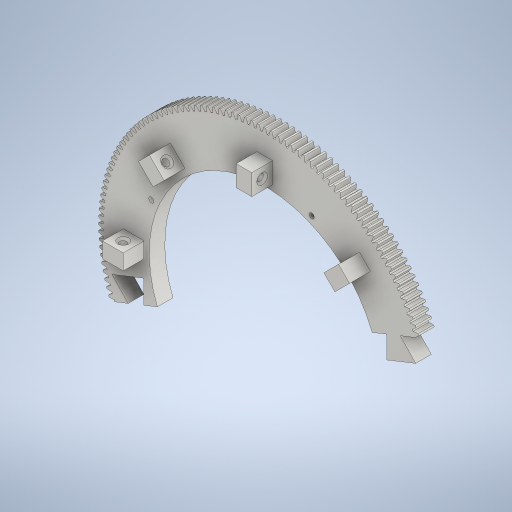
# Autodesk Inventor part: BearingGearMk2
Saved by Autodesk Inventor 2023 (Build 270158000, 158)
## iProperties
CustomPartVersion: 1
Created: 2023-04-03
Part Number: BearingGearMk2
Material: Steel
Document SubType Name: Modeling
Designer: czapa
Categories: <?xml version="1.0" encoding="UTF-16"?> <MemberInstance><Categories><FamilyTemplate><FamilyTemplateParameter ValueType="xs:double" Id="1" ObjectReferenceKey="da_z" ObjectType="kUserParameterObject"/><FamilyTemplateParameter ValueType="xs:double" Id="2" ObjectReferenceKey="da_b" ObjectType="kUserParameterObject"/><FamilyTemplateParameter ValueType="xs:double" Id="3" ObjectReferenceKey="da_beta" ObjectType="kUserParameterObject"/><FamilyTemplateParameter ValueType="xs:double" Id="4" ObjectReferenceKey="da_da" ObjectType="kUserParameterObject"/><FamilyTemplateParameter ValueType="xs:double" Id="5" ObjectReferenceKey="da_aw" ObjectType="kUserParameterObject"/><FamilyTemplateParameter ValueType="xs:string" Id="6" ObjectReferenceKey="EAIAABAAAACIAQAAAAAAAIAAAAAAAAAA" ObjectType="83910656" SubObjectId="SurfaceGeometry"/></FamilyTemplate><ParamToTemplateMap><ParamToTemplate CategoryParameter="//CategoryParameter[@InternalName='046C89C9-8512-4d59-83FE-43B91F4F132A']" TemplateParameter="1"/><ParamToTemplate CategoryParameter="//CategoryParameter[@InternalName='2552DF32-E462-4b46-AEBF-C6C7768E72AC']" TemplateParameter="2"/><ParamToTemplate CategoryParameter="//CategoryParameter[@InternalName='C9EE641D-15FC-4fae-A226-E94C4372FDD7']" TemplateParameter="3"/><ParamToTemplate><ParamToTemplate CategoryParameter="//CategoryParameter[@InternalName='00B6519A-459B-49c7-AD84-2E56D39A5744']" ConstantValue="-1.000000"/></ParamToTemplate><ParamToTemplate><ParamToTemplate CategoryParameter="//CategoryParameter[@InternalName='04B31F0E-C7A6-4894-AA32-9629BEFACF47']" ConstantValue="1.000000"/></ParamToTemplate><ParamToTemplate><ParamToTemplate CategoryParameter="//CategoryParameter[@InternalName='43CBEC2E-7847-49e7-A936-2F7889FCB2D9']" ConstantValue="0.250000"/></ParamToTemplate><ParamToTemplate><ParamToTemplate CategoryParameter="//CategoryParameter[@InternalName='B1EFC894-105D-4ebd-86BF-FA20ED196853']" ConstantValue="0.350000"/></ParamToTemplate><ParamToTemplate><ParamToTemplate CategoryParameter="//CategoryParameter[@InternalName='51175063-3D10-4879-93E8-6246FE8B403D']" ConstantValue="2060000000.000000"/></ParamToTemplate><ParamToTemplate><ParamToTemplate CategoryParameter="//CategoryParameter[@InternalName='A3A52E27-4454-46a9-B0BD-C932399B70AF']" ConstantValue="0.300000"/></ParamToTemplate><ParamToTemplate><ParamToTemplate CategoryParameter="//CategoryParameter[@InternalName='91B76062-C214-41d9-B1B9-14D2AB99603D']" ConstantValue="0.200000"/></ParamToTemplate><ParamToTemplate><ParamToTemplate CategoryParameter="//CategoryParameter[@InternalName='374E806E-8B8A-4dda-A9AA-1039D6500AD2']" ConstantValue="5.000000"/></ParamToTemplate><ParamToTemplate><ParamToTemplate CategoryParameter="//CategoryParameter[@InternalName='2D373A89-B862-43d6-8D0B-0CBF12AB9F6C']" ConstantValue="0.349066"/></ParamToTemplate><ParamToTemplate CategoryParameter="//CategoryParameter[@InternalName='37777632-D6A2-4fac-9D53-DB8ACD95C989']" TemplateParameter="4"/><ParamToTemplate CategoryParameter="//CategoryParameter[@InternalName='FD1017F1-B727-4f7e-9707-0F86F1FF9423']" TemplateParameter="5"/><ParamToTemplate><ParamToTemplate CategoryParameter="//CategoryParameter[@InternalName='9E1B4470-B2D3-4ff1-B813-535BB4CDF51A']" ConstantValue="3520000.000000"/></ParamToTemplate><ParamToTemplate><ParamToTemplate CategoryParameter="//CategoryParameter[@InternalName='F8452263-BFF6-458c-9FB1-07C4B99E95CD']" ConstantValue="11400000.000000"/></ParamToTemplate><ParamToTemplate><ParamToTemplate CategoryParameter="//CategoryParameter[@InternalName='3E3BB259-FD49-497f-8171-6EBC954A3479']" ConstantValue="2.000000"/></ParamToTemplate><ParamToTemplate CategoryParameter="//CategoryParameter[@InternalName='27C3BAF2-7550-4e4b-AE2C-0DB134B7D9B7']" TemplateParameter="6"/></ParamToTemplateMap><Category DisplayName="Gear" InternalName="DC85795E-93AB-48d5-8EEE-5A27447B64BD" Mnemonic="Gear"><CategoryParameter DisplayName="z" InternalName="046C89C9-8512-4d59-83FE-43B91F4F132A" Mnemonic="z"/><CategoryParameter DisplayName="b" InternalName="2552DF32-E462-4b46-AEBF-C6C7768E72AC" Mnemonic="b"/><CategoryParameter DisplayName="||b|" InternalName="C9EE641D-15FC-4fae-A226-E94C4372FDD7" Mnemonic="beta"/><CategoryParameter DisplayName="x" InternalName="00B6519A-459B-49c7-AD84-2E56D39A5744" Mnemonic="x"/><CategoryParameter DisplayName="a*" InternalName="04B31F0E-C7A6-4894-AA32-9629BEFACF47" Mnemonic="a"/><CategoryParameter DisplayName="c*" InternalName="43CBEC2E-7847-49e7-A936-2F7889FCB2D9" Mnemonic="c"/><CategoryParameter DisplayName="r|.f|*" InternalName="B1EFC894-105D-4ebd-86BF-FA20ED196853" Mnemonic="rf"/><CategoryParameter DisplayName="E" InternalName="51175063-3D10-4879-93E8-6246FE8B403D" Mnemonic="E"/><CategoryParameter DisplayName="||m|" InternalName="A3A52E27-4454-46a9-B0BD-C932399B70AF" Mnemonic="mi"/><Category DisplayName="SpurGear" InternalName="26C5A22E-A91E-4dfd-A3B3-23CCAFAE1764" Mnemonic="SpurGear"><CategoryParameter DisplayName="m" InternalName="91B76062-C214-41d9-B1B9-14D2AB99603D" Mnemonic="m"/><CategoryParameter DisplayName="P" InternalName="374E806E-8B8A-4dda-A9AA-1039D6500AD2" Mnemonic="PP"/><CategoryParameter DisplayName="||a|" InternalName="2D373A89-B862-43d6-8D0B-0CBF12AB9F6C" Mnemonic="alpha"/><CategoryParameter DisplayName="d|.a|" InternalName="37777632-D6A2-4fac-9D53-DB8ACD95C989" Mnemonic="da"/><CategoryParameter DisplayName="a|.w|" InternalName="FD1017F1-B727-4f7e-9707-0F86F1FF9423" Mnemonic="aw"/><CategoryParameter DisplayName="||s||.Flim|" InternalName="9E1B4470-B2D3-4ff1-B813-535BB4CDF51A" Mnemonic="sFlim"/><CategoryParameter DisplayName="||s||.Hlim|" InternalName="F8452263-BFF6-458c-9FB1-07C4B99E95CD" Mnemonic="sHlim"/><CategoryParameter DisplayName="type" InternalName="3E3BB259-FD49-497f-8171-6EBC954A3479" Mnemonic="type"/><CategoryParameter DisplayName="PitchDiameter" InternalName="27C3BAF2-7550-4e4b-AE2C-0DB134B7D9B7" Mnemonic="IDS_PITCHDIAM"/></Category></Category></Categories></MemberInstance>
Density: 1 g/cm^3
Appearance: Steel
Author: czapa
Autodesk Inventor part; units mm, degrees
(part 1 of 2)
ref_plane "YZ Plane" through (0, 0, 0) normal (1, 0, 0) x (0, 1, 0)
ref_plane "XZ Plane" through (0, 0, 0) normal (0, 1, 0) x (-1, 0, 0)
ref_plane "XY Plane" through (0, 0, 0) normal (0, 0, 1) x (1, 0, 0)
sketch "Sketch1" plane through (0, 0, 0) normal (0, 0, 1) x (1, 0, 0)
  circle A0 centre (0, 0) radius 160
  dimension "d0" = 320
  constraints: 1 centre point
  measures "d0" diameter of A0
extrude "Extrusion1" add sketch "Sketch1" along normal blind 15
ref_plane "Work Plane2" through (0, 0, 7.5) normal (0, 0, 1) x (1, 0, 0)
sketch "Sketch2" plane through (0, 0, 0) normal (0, 0, -1) x (-1, 0, 0)
  circle A0 centre (0, 0) radius 160 projected
  circle A1 centre (0, 0) radius 160
  dimension "d3" = 320
  constraints: 1 centre point, 1 coincident
  measures "d3" diameter of A1
surface extrude "Pitch Diameter" sketch "Sketch2" against normal through all shown no curves A1
ref_plane "Work Plane8" through (0, 0, 0) normal (0.9998072, 0.0196337, 0) x (0, 0, 1)
ref_plane "Work Plane9" through (0, 0, 0) normal (1, 0, 0) x (0, 1, 0)
spur gear teeth "Spur Gear" teeth 160 pitch diameter 320 tip diameter 320 root diameter 311 face width 20 start plane through (0, 0, 0) normal (0, 0, -1) x (-1, 0, 0)
sketch "Sketch3" plane through (0, 0, 15) normal (0, 0, 1) x (1, 0, 0)
  circle A0 centre (0, 0) radius 125
  circle A1 centre (0, 0) radius 111.25
  dimension "d49" = 250
  dimension "d50" = 222.5
  constraints: 2 centre point, 2 coincident
  measures "d49" diameter of A0
  measures "d50" diameter of A1
extrude "Extrusion2" cut sketch "Sketch3" against normal blind 15 contours A1
sketch "Sketch7" plane through (0, 0, 15) normal (0, 0, 1) x (1, 0, 0)
  line L0 (0, 116.25) -> (7.5, 116.25)
  line L1 (7.5, 116.25) -> (7.5, 136.25)
  line L2 (7.5, 116.25) -> (-7.5, 116.25)
  line L3 (-7.5, 116.25) -> (-7.5, 136.25)
  line L4 (-7.5, 136.25) -> (7.5, 136.25)
  line L5 (7.5, 136.25) -> (7.5, 116.25)
  line L6 (0, 0) -> (111.25, 0) construction
  circle A0 centre (0, 0) radius 111.25 projected
  point P0 (7.5, 136.25)
  point P1 (0, 111.25)
  dimension "d75" = 7.5
  dimension "d76" = 20
  dimension "d77" = 15
  dimension "d78" = 20
  dimension "d110" = 5
  constraints: 14 end point, 2 horizontal, 2 parallel, 2 perpendicular, 1 midpoint, 1 point on circle
  measures "d75" distance of L0.start L0.end
  measures "d76" distance of L0.end L1.end
  measures "d77" distance of L3.end L4.end
  measures "d78" distance of L2.end L3.end
  measures "d110" distance of A0.end point (0, 116.25)
extrude "Extrusion4" add sketch "Sketch7" along normal blind 20 contours L2 L3 L4 L1 L0
sketch "Sketch8" plane through (7.5, 116.25, 15) normal (1, 0, 0) x (0, 0, -1)
  line L0 (-20, 20) -> (-20, 0) projected
  line L1 (-20, 10) -> (-10, 10)
  line L2 (0, 20) -> (-20, 20) projected
  circle A0 centre (-10, 10) radius 3.25
  point P0 (15, -116.25)
  dimension "d81" = 6.5
  constraints: 2 end point, 1 centre point, 1 coincident, 1 midpoint, 1 parallel
  measures "d81" diameter of A0
extrude "Extrusion5" cut sketch "Sketch8" against normal blind 20
chamfer "Chamfer1" distance 2 angle 45 2 edges at (-7.5, 126.25, 28.25) (7.5, 126.25, 28.25)
pattern_circular "Circular Pattern3" count 8 over 360 about axis through (0, 0, 15) along (0, 0, -1) of "Extrusion4", "Extrusion5", "Chamfer1"
sketch "Sketch10" plane through (0, 0, 15) normal (0, 0, 1) x (1, 0, 0)
  circle A0 centre (0, 0) radius 118.125
  line L0 (0, 0) -> (45.2045, 109.1333)
  line L1 (0, 0) -> (118.125, 0) construction
  dimension "d111" = 67.5
  constraints: 4 end point, 2 coincident, 1 equal length, 1 horizontal, 3 other
  measures "d111" angle of L1 L0
hole "Hole2" at (45.2045, 109.1333, 15) direction (0, 0, -1) diameter 5 end through all
pattern_circular "Circular Pattern4" count 4 over 360 about axis through (0, 0, 15) along (0, 0, -1) of "Hole2"
sketch "Sketch11" plane through (0, 0, 15) normal (0, 0, 1) x (1, 0, 0)
  circle A0 centre (0, 0) radius 111.25 projected
  line L0 (0, 0) -> (111.25, 0) construction
  arc A1 (148.1195, 60.503) -> (147.5184, 61.9542) centre (0, 0) ccw projected
  line L1 (0, 0) -> (144.524, 57.3853)
  line L2 (0, 0) -> (3.1399, -7.9077)
  line L3 (0, 0) -> (-144.524, -57.3853)
  arc A2 (-144.524, -57.3853) -> (-148.1195, -60.503) centre (-126.4791, -81.8277) ccw projected
  line L4 (-144.524, -57.3853) -> (-123.9607, -49.2203)
  line L5 (-123.9607, -49.2203) -> (-116.5799, -67.8086)
  line L6 (-116.5799, -67.8086) -> (-102.6387, -62.2731)
  line L7 (-102.6387, -62.2731) -> (-117.4002, -46.6154)
  line L8 (-123.9607, -49.2203) -> (-131.3414, -30.632)
  line L9 (-117.4002, -25.0965) -> (-117.4002, -46.6154)
  line L10 (-117.4002, -46.6154) -> (-116.4708, -46.2464)
  line L11 (-117.4002, -25.0965) -> (-117.7692, -24.1671)
  line L12 (-117.7692, -24.1671) -> (-114.0516, -22.6909)
  line L13 (-116.4708, -23.6515) -> (-116.4708, -46.2464)
  line L14 (-145.2826, -36.1676) -> (-130.5212, -51.8253)
  line L15 (-145.2826, -36.1676) -> (-145.6517, -35.2382)
  line L16 (-145.6517, -35.2382) -> (-149.3693, -36.7143)
  line L17 (-146.9501, -35.7538) -> (-131.4506, -52.1943)
  line L18 (-145.6517, -35.2382) -> (-117.7692, -24.1671)
  line L19 (-116.5799, -67.8086) -> (-130.5212, -73.3442)
  line L20 (-130.5212, -73.3442) -> (-130.5212, -51.8253)
  line L21 (123.9607, 49.2203) -> (131.3414, 30.632)
  line L22 (131.3414, 30.632) -> (117.4002, 25.0965)
  line L23 (117.4002, 25.0965) -> (117.4002, 46.6154)
  line L24 (145.2826, 36.1676) -> (130.5212, 51.8253)
  line L25 (131.3414, 30.632) -> (145.2826, 36.1676)
  circle A3 centre (-109.1333, 45.2045) radius 2.5 projected
  circle A4 centre (-45.2045, -109.1333) radius 2.5 projected
  circle A5 centre (109.1333, -45.2045) radius 2.5 projected
  circle A6 centre (45.2045, 109.1333) radius 2.5 projected
  line L26 (-101.6466, 91.04) -> (-91.04, 101.6466) projected
  line L27 (-91.04, 101.6466) -> (-76.8979, 87.5045) projected
  line L28 (-76.8979, 87.5045) -> (-87.5045, 76.8979) projected
  line L29 (-87.5045, 76.8979) -> (-101.6466, 91.04) projected
  line L30 (-136.25, -7.5) -> (-136.25, 7.5) projected
  line L31 (-136.25, 7.5) -> (-116.25, 7.5) projected
  line L32 (-116.25, 7.5) -> (-116.25, -7.5) projected
  line L33 (-116.25, -7.5) -> (-136.25, -7.5) projected
  line L34 (-91.04, -101.6466) -> (-101.6466, -91.04) projected
  line L35 (-101.6466, -91.04) -> (-87.5045, -76.8979) projected
  line L36 (-87.5045, -76.8979) -> (-76.8979, -87.5045) projected
  line L37 (-76.8979, -87.5045) -> (-91.04, -101.6466) projected
  line L38 (7.5, -136.25) -> (-7.5, -136.25) projected
  line L39 (-7.5, -136.25) -> (-7.5, -116.25) projected
  line L40 (-7.5, -116.25) -> (7.5, -116.25) projected
  line L41 (7.5, -116.25) -> (7.5, -136.25) projected
  line L42 (101.6466, -91.04) -> (91.04, -101.6466) projected
  line L43 (91.04, -101.6466) -> (76.8979, -87.5045) projected
  line L44 (76.8979, -87.5045) -> (87.5045, -76.8979) projected
  line L45 (87.5045, -76.8979) -> (101.6466, -91.04) projected
  line L46 (136.25, 7.5) -> (136.25, -7.5) projected
  line L47 (136.25, -7.5) -> (116.25, -7.5) projected
  line L48 (116.25, -7.5) -> (116.25, 7.5) projected
  line L49 (116.25, 7.5) -> (136.25, 7.5) projected
  line L50 (91.04, 101.6466) -> (101.6466, 91.04) projected
  line L51 (101.6466, 91.04) -> (87.5045, 76.8979) projected
  line L52 (87.5045, 76.8979) -> (76.8979, 87.5045) projected
  line L53 (76.8979, 87.5045) -> (91.04, 101.6466) projected
  line L54 (-7.5, 136.25) -> (7.5, 136.25) projected
  line L55 (7.5, 136.25) -> (7.5, 116.25) projected
  line L56 (7.5, 116.25) -> (-7.5, 116.25) projected
  line L57 (-7.5, 116.25) -> (-7.5, 136.25) projected
  circle A7 centre (0, 0) radius 111.25 projected
  arc A8 (-7.0663, 159.8439) -> (-8.3923, 155.2734) centre (21.3596, 149.1191) ccw projected
  arc A9 (-8.3923, 155.2734) -> (-9.9163, 155.1835) centre (0, 0) ccw projected
  arc A10 (-9.9163, 155.1835) -> (-11.7703, 159.5665) centre (-38.7386, 145.575) ccw projected
  arc A11 (-11.7703, 159.5665) -> (-13.3363, 159.4432) centre (0, 0) ccw projected
  arc A12 (-13.3363, 159.4432) -> (-14.4819, 154.8242) centre (15.4887, 149.8427) ccw projected
  arc A13 (-14.4819, 154.8242) -> (-16.0011, 154.6745) centre (0, 0) ccw projected
  arc A14 (-16.0011, 154.6745) -> (-18.0258, 158.9814) centre (-44.424, 143.9419) ccw projected
  arc A15 (-18.0258, 158.9814) -> (-19.5857, 158.7967) centre (0, 0) ccw projected
  arc A16 (-19.5857, 158.7967) -> (-20.5491, 154.1363) centre (9.594, 150.3353) ccw projected
  arc A17 (-20.5491, 154.1363) -> (-22.0613, 153.9271) centre (0, 0) ccw projected
  arc A18 (-22.0613, 153.9271) -> (-24.2535, 158.1511) centre (-50.0409, 142.0868) ccw projected
  arc A19 (-24.2535, 158.1511) -> (-25.8049, 157.9054) centre (0, 0) ccw projected
  arc A20 (-25.8049, 157.9054) -> (-26.5846, 153.2107) centre (3.6845, 150.5961) ccw projected
  arc A21 (-26.5846, 153.2107) -> (-28.0874, 152.9423) centre (0, 0) ccw projected
  arc A22 (-28.0874, 152.9423) -> (-30.4438, 157.077) centre (-55.5806, 140.0127) ccw projected
  arc A23 (-30.4438, 157.077) -> (-31.9844, 156.7705) centre (0, 0) ccw projected
  arc A24 (-31.9844, 156.7705) -> (-32.5791, 152.0488) centre (-2.2308, 150.6246) ccw projected
  arc A25 (-32.5791, 152.0488) -> (-34.0702, 151.7217) centre (0, 0) ccw projected
  arc A26 (-34.0702, 151.7217) -> (-36.5871, 155.7607) centre (-61.0346, 137.7226) ccw projected
  arc A27 (-36.5871, 155.7607) -> (-38.1145, 155.394) centre (0, 0) ccw projected
  arc A28 (-38.1145, 155.394) -> (-38.5234, 150.6526) centre (-8.1425, 150.4209) ccw projected
  arc A29 (-38.5234, 150.6526) -> (-40.0005, 150.2671) centre (0, 0) ccw projected
  arc A30 (-40.0005, 150.2671) -> (-42.674, 154.2042) centre (-66.3945, 135.2203) ccw projected
  arc A31 (-42.674, 154.2042) -> (-44.1859, 153.7778) centre (0, 0) ccw projected
  arc A32 (-44.1859, 153.7778) -> (-44.4083, 149.024) centre (-14.0418, 149.9853) ccw projected
  arc A33 (-44.4083, 149.024) -> (-45.8692, 148.5809) centre (0, 0) ccw projected
  arc A34 (-45.8692, 148.5809) -> (-48.6952, 152.4099) centre (-71.6521, 132.5094) ccw projected
  arc A35 (-48.6952, 152.4099) -> (-50.1891, 151.9245) centre (0, 0) ccw projected
  arc A36 (-50.1891, 151.9245) -> (-50.2247, 147.1657) centre (-19.9193, 149.3183) ccw projected
  arc A37 (-50.2247, 147.1657) -> (-51.6671, 146.6655) centre (0, 0) ccw projected
  arc A38 (-51.6671, 146.6655) -> (-54.6412, 150.3806) centre (-76.7991, 129.5942) ccw projected
  arc A39 (-54.6412, 150.3806) -> (-56.1149, 149.837) centre (0, 0) ccw projected
  arc A40 (-56.1149, 149.837) -> (-55.9637, 145.0804) centre (-25.7662, 148.4212) ccw projected
  arc A41 (-55.9637, 145.0804) -> (-57.3853, 144.524) centre (0, 0) ccw projected
  arc A42 (-57.3853, 144.524) -> (-60.503, 148.1195) centre (-81.8277, 126.4791) ccw projected
  arc A43 (-60.503, 148.1195) -> (-61.9542, 147.5184) centre (0, 0) ccw projected
  arc A44 (-61.9542, 147.5184) -> (-61.6164, 142.7714) centre (-31.5733, 147.2952) ccw projected
  arc A45 (-61.6164, 142.7714) -> (-63.015, 142.1596) centre (0, 0) ccw projected
  arc A46 (-63.015, 142.1596) -> (-66.2715, 145.63) centre (-86.7302, 123.1691) ccw projected
  arc A47 (-66.2715, 145.63) -> (-67.698, 144.9723) centre (0, 0) ccw projected
  arc A48 (-67.698, 144.9723) -> (-67.174, 140.2423) centre (-37.3317, 145.9421) ccw projected
  arc A49 (-67.174, 140.2423) -> (-68.5476, 139.5761) centre (0, 0) ccw projected
  arc A50 (-68.5476, 139.5761) -> (-71.9378, 142.9159) centre (-91.4989, 119.6691) ccw projected
  arc A51 (-71.9378, 142.9159) -> (-73.3374, 142.2028) centre (0, 0) ccw projected
  arc A52 (-73.3374, 142.2028) -> (-72.6281, 137.4969) centre (-43.0326, 144.3639) ccw projected
  arc A53 (-72.6281, 137.4969) -> (-73.9745, 136.7773) centre (0, 0) ccw projected
  arc A54 (-73.9745, 136.7773) -> (-77.4932, 139.9814) centre (-96.1266, 115.9846) ccw projected
  arc A55 (-77.4932, 139.9814) -> (-78.8637, 139.2139) centre (0, 0) ccw projected
  arc A56 (-78.8637, 139.2139) -> (-77.9702, 134.5396) centre (-48.6671, 142.5632) ccw projected
  arc A57 (-77.9702, 134.5396) -> (-79.2873, 133.7676) centre (0, 0) ccw projected
  arc A58 (-79.2873, 133.7676) -> (-82.9291, 136.8312) centre (-100.606, 112.1213) ccw projected
  arc A59 (-82.9291, 136.8312) -> (-84.2684, 136.0104) centre (0, 0) ccw projected
  arc A60 (-84.2684, 136.0104) -> (-83.1921, 131.3747) centre (-54.2266, 140.5426) ccw projected
  arc A61 (-83.1921, 131.3747) -> (-84.4779, 130.5517) centre (0, 0) ccw projected
  arc A62 (-84.4779, 130.5517) -> (-88.2371, 133.4699) centre (-104.9303, 108.0851) ccw projected
  arc A63 (-88.2371, 133.4699) -> (-89.5432, 132.5972) centre (0, 0) ccw projected
  arc A64 (-89.5432, 132.5972) -> (-88.2857, 128.0073) centre (-59.7025, 138.3053) ccw projected
  arc A65 (-88.2857, 128.0073) -> (-89.5382, 127.1344) centre (0, 0) ccw projected
  arc A66 (-89.5382, 127.1344) -> (-93.4091, 129.9028) centre (-109.0928, 103.8822) ccw projected
  arc A67 (-93.4091, 129.9028) -> (-94.6799, 128.9795) centre (0, 0) ccw projected
  arc A68 (-94.6799, 128.9795) -> (-93.2432, 124.4426) centre (-65.0863, 135.8548) ccw projected
  arc A69 (-93.2432, 124.4426) -> (-94.4604, 123.5212) centre (0, 0) ccw projected
  arc A70 (-94.4604, 123.5212) -> (-98.4371, 126.1354) centre (-113.0871, 99.5191) ccw projected
  arc A71 (-98.4371, 126.1354) -> (-99.6706, 125.163) centre (0, 0) ccw projected
  arc A72 (-99.6706, 125.163) -> (-98.0569, 120.6859) centre (-70.3698, 133.1948) ccw projected
  arc A73 (-98.0569, 120.6859) -> (-99.237, 119.7174) centre (0, 0) ccw projected
  arc A74 (-99.237, 119.7174) -> (-103.3132, 122.1736) centre (-116.907, 95.0026) ccw projected
  arc A75 (-103.3132, 122.1736) -> (-104.5077, 121.1534) centre (0, 0) ccw projected
  arc A76 (-104.5077, 121.1534) -> (-102.7194, 116.7432) centre (-75.5447, 130.3294) ccw projected
  arc A77 (-102.7194, 116.7432) -> (-103.8606, 115.7291) centre (0, 0) ccw projected
  arc A78 (-103.8606, 115.7291) -> (-108.0301, 118.0233) centre (-120.5467, 90.3396) ccw projected
  arc A79 (-108.0301, 118.0233) -> (-109.1835, 116.9571) centre (0, 0) ccw projected
  arc A80 (-109.1835, 116.9571) -> (-107.2236, 112.6204) centre (-80.6032, 127.263) ccw projected
  arc A81 (-107.2236, 112.6204) -> (-108.324, 111.5623) centre (0, 0) ccw projected
  arc A82 (-108.324, 111.5623) -> (-112.5804, 113.6911) centre (-124.0004, 85.5374) ccw projected
  arc A83 (-112.5804, 113.6911) -> (-113.6911, 112.5804) centre (0, 0) ccw projected
  arc A84 (-113.6911, 112.5804) -> (-111.5623, 108.324) centre (-85.5374, 124.0004) ccw projected
  arc A85 (-111.5623, 108.324) -> (-112.6204, 107.2236) centre (0, 0) ccw projected
  arc A86 (-112.6204, 107.2236) -> (-116.9571, 109.1835) centre (-127.263, 80.6032) ccw projected
  arc A87 (-116.9571, 109.1835) -> (-118.0233, 108.0301) centre (0, 0) ccw projected
  arc A88 (-118.0233, 108.0301) -> (-115.7291, 103.8606) centre (-90.3396, 120.5467) ccw projected
  arc A89 (-115.7291, 103.8606) -> (-116.7432, 102.7194) centre (0, 0) ccw projected
  arc A90 (-116.7432, 102.7194) -> (-121.1534, 104.5077) centre (-130.3294, 75.5447) ccw projected
  arc A91 (-121.1534, 104.5077) -> (-122.1736, 103.3132) centre (0, 0) ccw projected
  arc A92 (-122.1736, 103.3132) -> (-119.7174, 99.237) centre (-95.0026, 116.907) ccw projected
  arc A93 (-119.7174, 99.237) -> (-120.6859, 98.0569) centre (0, 0) ccw projected
  arc A94 (-120.6859, 98.0569) -> (-125.163, 99.6706) centre (-133.1948, 70.3698) ccw projected
  arc A95 (-125.163, 99.6706) -> (-126.1354, 98.4371) centre (0, 0) ccw projected
  arc A96 (-126.1354, 98.4371) -> (-123.5212, 94.4604) centre (-99.5191, 113.0871) ccw projected
  arc A97 (-123.5212, 94.4604) -> (-124.4426, 93.2432) centre (0, 0) ccw projected
  arc A98 (-124.4426, 93.2432) -> (-128.9795, 94.6799) centre (-135.8548, 65.0863) ccw projected
  arc A99 (-128.9795, 94.6799) -> (-129.9028, 93.4091) centre (0, 0) ccw projected
  arc A100 (-129.9028, 93.4091) -> (-127.1344, 89.5382) centre (-103.8822, 109.0928) ccw projected
  arc A101 (-127.1344, 89.5382) -> (-128.0073, 88.2857) centre (0, 0) ccw projected
  arc A102 (-128.0073, 88.2857) -> (-132.5972, 89.5432) centre (-138.3053, 59.7025) ccw projected
  arc A103 (-132.5972, 89.5432) -> (-133.4699, 88.2371) centre (0, 0) ccw projected
  arc A104 (-133.4699, 88.2371) -> (-130.5517, 84.4779) centre (-108.0851, 104.9303) ccw projected
  arc A105 (-130.5517, 84.4779) -> (-131.3747, 83.1921) centre (0, 0) ccw projected
  arc A106 (-131.3747, 83.1921) -> (-136.0104, 84.2684) centre (-140.5426, 54.2266) ccw projected
  arc A107 (-136.0104, 84.2684) -> (-136.8312, 82.9291) centre (0, 0) ccw projected
  arc A108 (-136.8312, 82.9291) -> (-133.7676, 79.2873) centre (-112.1213, 100.606) ccw projected
  arc A109 (-133.7676, 79.2873) -> (-134.5396, 77.9702) centre (0, 0) ccw projected
  arc A110 (-134.5396, 77.9702) -> (-139.2139, 78.8637) centre (-142.5632, 48.6671) ccw projected
  arc A111 (-139.2139, 78.8637) -> (-139.9814, 77.4932) centre (0, 0) ccw projected
  arc A112 (-139.9814, 77.4932) -> (-136.7773, 73.9745) centre (-115.9846, 96.1266) ccw projected
  arc A113 (-136.7773, 73.9745) -> (-137.4969, 72.6281) centre (0, 0) ccw projected
  arc A114 (-137.4969, 72.6281) -> (-142.2028, 73.3374) centre (-144.3639, 43.0326) ccw projected
  arc A115 (-142.2028, 73.3374) -> (-142.9159, 71.9378) centre (0, 0) ccw projected
  arc A116 (-142.9159, 71.9378) -> (-139.5761, 68.5476) centre (-119.6691, 91.4989) ccw projected
  arc A117 (-139.5761, 68.5476) -> (-140.2423, 67.174) centre (0, 0) ccw projected
  arc A118 (-140.2423, 67.174) -> (-144.9723, 67.698) centre (-145.9421, 37.3317) ccw projected
  arc A119 (-144.9723, 67.698) -> (-145.63, 66.2715) centre (0, 0) ccw projected
  arc A120 (-145.63, 66.2715) -> (-142.1596, 63.015) centre (-123.1691, 86.7302) ccw projected
  arc A121 (-142.1596, 63.015) -> (-142.7714, 61.6164) centre (0, 0) ccw projected
  arc A122 (-142.7714, 61.6164) -> (-147.5184, 61.9542) centre (-147.2952, 31.5733) ccw projected
  arc A123 (-147.5184, 61.9542) -> (-148.1195, 60.503) centre (0, 0) ccw projected
  arc A124 (-148.1195, 60.503) -> (-144.524, 57.3853) centre (-126.4791, 81.8277) ccw projected
  arc A125 (-144.524, 57.3853) -> (-145.0804, 55.9637) centre (0, 0) ccw projected
  arc A126 (-145.0804, 55.9637) -> (-149.837, 56.1149) centre (-148.4212, 25.7662) ccw projected
  arc A127 (-149.837, 56.1149) -> (-150.3806, 54.6412) centre (0, 0) ccw projected
  arc A128 (-150.3806, 54.6412) -> (-146.6655, 51.6671) centre (-129.5942, 76.7991) ccw projected
  arc A129 (-146.6655, 51.6671) -> (-147.1657, 50.2247) centre (0, 0) ccw projected
  arc A130 (-147.1657, 50.2247) -> (-151.9245, 50.1891) centre (-149.3183, 19.9193) ccw projected
  arc A131 (-151.9245, 50.1891) -> (-152.4099, 48.6952) centre (0, 0) ccw projected
  arc A132 (-152.4099, 48.6952) -> (-148.5809, 45.8692) centre (-132.5094, 71.6521) ccw projected
  arc A133 (-148.5809, 45.8692) -> (-149.024, 44.4083) centre (0, 0) ccw projected
  arc A134 (-149.024, 44.4083) -> (-153.7778, 44.1859) centre (-149.9853, 14.0418) ccw projected
  arc A135 (-153.7778, 44.1859) -> (-154.2042, 42.674) centre (0, 0) ccw projected
  arc A136 (-154.2042, 42.674) -> (-150.2671, 40.0005) centre (-135.2203, 66.3945) ccw projected
  arc A137 (-150.2671, 40.0005) -> (-150.6526, 38.5234) centre (0, 0) ccw projected
  arc A138 (-150.6526, 38.5234) -> (-155.394, 38.1145) centre (-150.4209, 8.1425) ccw projected
  arc A139 (-155.394, 38.1145) -> (-155.7607, 36.5871) centre (0, 0) ccw projected
  arc A140 (-155.7607, 36.5871) -> (-151.7217, 34.0702) centre (-137.7226, 61.0346) ccw projected
  arc A141 (-151.7217, 34.0702) -> (-152.0488, 32.5791) centre (0, 0) ccw projected
  arc A142 (-152.0488, 32.5791) -> (-156.7705, 31.9844) centre (-150.6246, 2.2308) ccw projected
  arc A143 (-156.7705, 31.9844) -> (-157.077, 30.4438) centre (0, 0) ccw projected
  arc A144 (-157.077, 30.4438) -> (-152.9423, 28.0874) centre (-140.0127, 55.5806) ccw projected
  arc A145 (-152.9423, 28.0874) -> (-153.2107, 26.5846) centre (0, 0) ccw projected
  arc A146 (-153.2107, 26.5846) -> (-157.9054, 25.8049) centre (-150.5961, -3.6845) ccw projected
  arc A147 (-157.9054, 25.8049) -> (-158.1511, 24.2535) centre (0, 0) ccw projected
  arc A148 (-158.1511, 24.2535) -> (-153.9271, 22.0613) centre (-142.0868, 50.0409) ccw projected
  arc A149 (-153.9271, 22.0613) -> (-154.1363, 20.5491) centre (0, 0) ccw projected
  arc A150 (-154.1363, 20.5491) -> (-158.7967, 19.5857) centre (-150.3353, -9.594) ccw projected
  arc A151 (-158.7967, 19.5857) -> (-158.9814, 18.0258) centre (0, 0) ccw projected
  arc A152 (-158.9814, 18.0258) -> (-154.6745, 16.0011) centre (-143.9419, 44.424) ccw projected
  arc A153 (-154.6745, 16.0011) -> (-154.8242, 14.4819) centre (0, 0) ccw projected
  arc A154 (-154.8242, 14.4819) -> (-159.4432, 13.3363) centre (-149.8427, -15.4887) ccw projected
  arc A155 (-159.4432, 13.3363) -> (-159.5665, 11.7703) centre (0, 0) ccw projected
  arc A156 (-159.5665, 11.7703) -> (-155.1835, 9.9163) centre (-145.575, 38.7386) ccw projected
  arc A157 (-155.1835, 9.9163) -> (-155.2734, 8.3923) centre (0, 0) ccw projected
  arc A158 (-155.2734, 8.3923) -> (-159.8439, 7.0663) centre (-149.1191, -21.3596) ccw projected
  arc A159 (-159.8439, 7.0663) -> (-159.9056, 5.4967) centre (0, 0) ccw projected
  arc A160 (-159.9056, 5.4967) -> (-155.4532, 3.8162) centre (-146.9836, 32.9935) ccw projected
  arc A161 (-155.4532, 3.8162) -> (-155.4831, 2.2898) centre (0, 0) ccw projected
  arc A162 (-155.4831, 2.2898) -> (-159.9981, 0.7854) centre (-148.1656, -27.1975) ccw projected
  arc A163 (-159.9981, 0.7854) -> (-159.9981, -0.7854) centre (0, 0) ccw projected
  arc A164 (-159.9981, -0.7854) -> (-155.4831, -2.2898) centre (-148.1656, 27.1975) ccw projected
  arc A165 (-155.4831, -2.2898) -> (-155.4532, -3.8162) centre (0, 0) ccw projected
  arc A166 (-155.4532, -3.8162) -> (-159.9056, -5.4967) centre (-146.9836, -32.9935) ccw projected
  arc A167 (-159.9056, -5.4967) -> (-159.8439, -7.0663) centre (0, 0) ccw projected
  arc A168 (-159.8439, -7.0663) -> (-155.2734, -8.3923) centre (-149.1191, 21.3596) ccw projected
  arc A169 (-155.2734, -8.3923) -> (-155.1835, -9.9163) centre (0, 0) ccw projected
  arc A170 (-155.1835, -9.9163) -> (-159.5665, -11.7703) centre (-145.575, -38.7386) ccw projected
  arc A171 (-159.5665, -11.7703) -> (-159.4432, -13.3363) centre (0, 0) ccw projected
  arc A172 (-159.4432, -13.3363) -> (-154.8242, -14.4819) centre (-149.8427, 15.4887) ccw projected
  arc A173 (-154.8242, -14.4819) -> (-154.6745, -16.0011) centre (0, 0) ccw projected
  arc A174 (-154.6745, -16.0011) -> (-158.9814, -18.0258) centre (-143.9419, -44.424) ccw projected
  arc A175 (-158.9814, -18.0258) -> (-158.7967, -19.5857) centre (0, 0) ccw projected
  arc A176 (-158.7967, -19.5857) -> (-154.1363, -20.5491) centre (-150.3353, 9.594) ccw projected
  arc A177 (-154.1363, -20.5491) -> (-153.9271, -22.0613) centre (0, 0) ccw projected
  arc A178 (-153.9271, -22.0613) -> (-158.1511, -24.2535) centre (-142.0868, -50.0409) ccw projected
  arc A179 (-158.1511, -24.2535) -> (-157.9054, -25.8049) centre (0, 0) ccw projected
  arc A180 (-157.9054, -25.8049) -> (-153.2107, -26.5846) centre (-150.5961, 3.6845) ccw projected
  arc A181 (-153.2107, -26.5846) -> (-152.9423, -28.0874) centre (0, 0) ccw projected
  arc A182 (-152.9423, -28.0874) -> (-157.077, -30.4438) centre (-140.0127, -55.5806) ccw projected
  arc A183 (-157.077, -30.4438) -> (-156.7705, -31.9844) centre (0, 0) ccw projected
  arc A184 (-156.7705, -31.9844) -> (-152.0488, -32.5791) centre (-150.6246, -2.2308) ccw projected
  arc A185 (-152.0488, -32.5791) -> (-151.7217, -34.0702) centre (0, 0) ccw projected
  arc A186 (-151.7217, -34.0702) -> (-155.7607, -36.5871) centre (-137.7226, -61.0346) ccw projected
  arc A187 (-155.7607, -36.5871) -> (-155.394, -38.1145) centre (0, 0) ccw projected
  arc A188 (-155.394, -38.1145) -> (-150.6526, -38.5234) centre (-150.4209, -8.1425) ccw projected
  arc A189 (-150.6526, -38.5234) -> (-150.2671, -40.0005) centre (0, 0) ccw projected
  arc A190 (-150.2671, -40.0005) -> (-154.2042, -42.674) centre (-135.2203, -66.3945) ccw projected
  arc A191 (-154.2042, -42.674) -> (-153.7778, -44.1859) centre (0, 0) ccw projected
  arc A192 (-153.7778, -44.1859) -> (-149.024, -44.4083) centre (-149.9853, -14.0418) ccw projected
  arc A193 (-149.024, -44.4083) -> (-148.5809, -45.8692) centre (0, 0) ccw projected
  arc A194 (-148.5809, -45.8692) -> (-152.4099, -48.6952) centre (-132.5094, -71.6521) ccw projected
  arc A195 (-152.4099, -48.6952) -> (-151.9245, -50.1891) centre (0, 0) ccw projected
  arc A196 (-151.9245, -50.1891) -> (-147.1657, -50.2247) centre (-149.3183, -19.9193) ccw projected
  arc A197 (-147.1657, -50.2247) -> (-146.6655, -51.6671) centre (0, 0) ccw projected
  arc A198 (-146.6655, -51.6671) -> (-150.3806, -54.6412) centre (-129.5942, -76.7991) ccw projected
  arc A199 (-150.3806, -54.6412) -> (-149.837, -56.1149) centre (0, 0) ccw projected
  arc A200 (-149.837, -56.1149) -> (-145.0804, -55.9637) centre (-148.4212, -25.7662) ccw projected
  arc A201 (-145.0804, -55.9637) -> (-144.524, -57.3853) centre (0, 0) ccw projected
  arc A202 (-144.524, -57.3853) -> (-148.1195, -60.503) centre (-126.4791, -81.8277) ccw projected
  arc A203 (-148.1195, -60.503) -> (-147.5184, -61.9542) centre (0, 0) ccw projected
  arc A204 (-147.5184, -61.9542) -> (-142.7714, -61.6164) centre (-147.2952, -31.5733) ccw projected
  arc A205 (-142.7714, -61.6164) -> (-142.1596, -63.015) centre (0, 0) ccw projected
  arc A206 (-142.1596, -63.015) -> (-145.63, -66.2715) centre (-123.1691, -86.7302) ccw projected
  arc A207 (-145.63, -66.2715) -> (-144.9723, -67.698) centre (0, 0) ccw projected
  arc A208 (-144.9723, -67.698) -> (-140.2423, -67.174) centre (-145.9421, -37.3317) ccw projected
  arc A209 (-140.2423, -67.174) -> (-139.5761, -68.5476) centre (0, 0) ccw projected
  arc A210 (-139.5761, -68.5476) -> (-142.9159, -71.9378) centre (-119.6691, -91.4989) ccw projected
  arc A211 (-142.9159, -71.9378) -> (-142.2028, -73.3374) centre (0, 0) ccw projected
  arc A212 (-142.2028, -73.3374) -> (-137.4969, -72.6281) centre (-144.3639, -43.0326) ccw projected
  arc A213 (-137.4969, -72.6281) -> (-136.7773, -73.9745) centre (0, 0) ccw projected
  arc A214 (-136.7773, -73.9745) -> (-139.9814, -77.4932) centre (-115.9846, -96.1266) ccw projected
  arc A215 (-139.9814, -77.4932) -> (-139.2139, -78.8637) centre (0, 0) ccw projected
  arc A216 (-139.2139, -78.8637) -> (-134.5396, -77.9702) centre (-142.5632, -48.6671) ccw projected
  arc A217 (-134.5396, -77.9702) -> (-133.7676, -79.2873) centre (0, 0) ccw projected
  arc A218 (-133.7676, -79.2873) -> (-136.8312, -82.9291) centre (-112.1213, -100.606) ccw projected
  arc A219 (-136.8312, -82.9291) -> (-136.0104, -84.2684) centre (0, 0) ccw projected
  arc A220 (-136.0104, -84.2684) -> (-131.3747, -83.1921) centre (-140.5426, -54.2266) ccw projected
  arc A221 (-131.3747, -83.1921) -> (-130.5517, -84.4779) centre (0, 0) ccw projected
  arc A222 (-130.5517, -84.4779) -> (-133.4699, -88.2371) centre (-108.0851, -104.9303) ccw projected
  arc A223 (-133.4699, -88.2371) -> (-132.5972, -89.5432) centre (0, 0) ccw projected
  arc A224 (-132.5972, -89.5432) -> (-128.0073, -88.2857) centre (-138.3053, -59.7025) ccw projected
  arc A225 (-128.0073, -88.2857) -> (-127.1344, -89.5382) centre (0, 0) ccw projected
  arc A226 (-127.1344, -89.5382) -> (-129.9028, -93.4091) centre (-103.8822, -109.0928) ccw projected
  arc A227 (-129.9028, -93.4091) -> (-128.9795, -94.6799) centre (0, 0) ccw projected
  arc A228 (-128.9795, -94.6799) -> (-124.4426, -93.2432) centre (-135.8548, -65.0863) ccw projected
  arc A229 (-124.4426, -93.2432) -> (-123.5212, -94.4604) centre (0, 0) ccw projected
  arc A230 (-123.5212, -94.4604) -> (-126.1354, -98.4371) centre (-99.5191, -113.0871) ccw projected
  arc A231 (-126.1354, -98.4371) -> (-125.163, -99.6706) centre (0, 0) ccw projected
  arc A232 (-125.163, -99.6706) -> (-120.6859, -98.0569) centre (-133.1948, -70.3698) ccw projected
  arc A233 (-120.6859, -98.0569) -> (-119.7174, -99.237) centre (0, 0) ccw projected
  arc A234 (-119.7174, -99.237) -> (-122.1736, -103.3132) centre (-95.0026, -116.907) ccw projected
  arc A235 (-122.1736, -103.3132) -> (-121.1534, -104.5077) centre (0, 0) ccw projected
  arc A236 (-121.1534, -104.5077) -> (-116.7432, -102.7194) centre (-130.3294, -75.5447) ccw projected
  arc A237 (-116.7432, -102.7194) -> (-115.7291, -103.8606) centre (0, 0) ccw projected
  arc A238 (-115.7291, -103.8606) -> (-118.0233, -108.0301) centre (-90.3396, -120.5467) ccw projected
  arc A239 (-118.0233, -108.0301) -> (-116.9571, -109.1835) centre (0, 0) ccw projected
  arc A240 (-116.9571, -109.1835) -> (-112.6204, -107.2236) centre (-127.263, -80.6032) ccw projected
  arc A241 (-112.6204, -107.2236) -> (-111.5623, -108.324) centre (0, 0) ccw projected
  arc A242 (-111.5623, -108.324) -> (-113.6911, -112.5804) centre (-85.5374, -124.0004) ccw projected
  arc A243 (-113.6911, -112.5804) -> (-112.5804, -113.6911) centre (0, 0) ccw projected
  arc A244 (-112.5804, -113.6911) -> (-108.324, -111.5623) centre (-124.0004, -85.5374) ccw projected
  arc A245 (-108.324, -111.5623) -> (-107.2236, -112.6204) centre (0, 0) ccw projected
  arc A246 (-107.2236, -112.6204) -> (-109.1835, -116.9571) centre (-80.6032, -127.263) ccw projected
  arc A247 (-109.1835, -116.9571) -> (-108.0301, -118.0233) centre (0, 0) ccw projected
  arc A248 (-108.0301, -118.0233) -> (-103.8606, -115.7291) centre (-120.5467, -90.3396) ccw projected
  arc A249 (-103.8606, -115.7291) -> (-102.7194, -116.7432) centre (0, 0) ccw projected
  arc A250 (-102.7194, -116.7432) -> (-104.5077, -121.1534) centre (-75.5447, -130.3294) ccw projected
  arc A251 (-104.5077, -121.1534) -> (-103.3132, -122.1736) centre (0, 0) ccw projected
  arc A252 (-103.3132, -122.1736) -> (-99.237, -119.7174) centre (-116.907, -95.0026) ccw projected
  arc A253 (-99.237, -119.7174) -> (-98.0569, -120.6859) centre (0, 0) ccw projected
  arc A254 (-98.0569, -120.6859) -> (-99.6706, -125.163) centre (-70.3698, -133.1948) ccw projected
  arc A255 (-99.6706, -125.163) -> (-98.4371, -126.1354) centre (0, 0) ccw projected
  arc A256 (-98.4371, -126.1354) -> (-94.4604, -123.5212) centre (-113.0871, -99.5191) ccw projected
  arc A257 (-94.4604, -123.5212) -> (-93.2432, -124.4426) centre (0, 0) ccw projected
  arc A258 (-93.2432, -124.4426) -> (-94.6799, -128.9795) centre (-65.0863, -135.8548) ccw projected
  arc A259 (-94.6799, -128.9795) -> (-93.4091, -129.9028) centre (0, 0) ccw projected
  arc A260 (-93.4091, -129.9028) -> (-89.5382, -127.1344) centre (-109.0928, -103.8822) ccw projected
  arc A261 (-89.5382, -127.1344) -> (-88.2857, -128.0073) centre (0, 0) ccw projected
  arc A262 (-88.2857, -128.0073) -> (-89.5432, -132.5972) centre (-59.7025, -138.3053) ccw projected
  arc A263 (-89.5432, -132.5972) -> (-88.2371, -133.4699) centre (0, 0) ccw projected
  arc A264 (-88.2371, -133.4699) -> (-84.4779, -130.5517) centre (-104.9303, -108.0851) ccw projected
  arc A265 (-84.4779, -130.5517) -> (-83.1921, -131.3747) centre (0, 0) ccw projected
  arc A266 (-83.1921, -131.3747) -> (-84.2684, -136.0104) centre (-54.2266, -140.5426) ccw projected
  arc A267 (-84.2684, -136.0104) -> (-82.9291, -136.8312) centre (0, 0) ccw projected
  arc A268 (-82.9291, -136.8312) -> (-79.2873, -133.7676) centre (-100.606, -112.1213) ccw projected
  arc A269 (-79.2873, -133.7676) -> (-77.9702, -134.5396) centre (0, 0) ccw projected
  arc A270 (-77.9702, -134.5396) -> (-78.8637, -139.2139) centre (-48.6671, -142.5632) ccw projected
  arc A271 (-78.8637, -139.2139) -> (-77.4932, -139.9814) centre (0, 0) ccw projected
  arc A272 (-77.4932, -139.9814) -> (-73.9745, -136.7773) centre (-96.1266, -115.9846) ccw projected
  arc A273 (-73.9745, -136.7773) -> (-72.6281, -137.4969) centre (0, 0) ccw projected
  arc A274 (-72.6281, -137.4969) -> (-73.3374, -142.2028) centre (-43.0326, -144.3639) ccw projected
  arc A275 (-73.3374, -142.2028) -> (-71.9378, -142.9159) centre (0, 0) ccw projected
  arc A276 (-71.9378, -142.9159) -> (-68.5476, -139.5761) centre (-91.4989, -119.6691) ccw projected
  arc A277 (-68.5476, -139.5761) -> (-67.174, -140.2423) centre (0, 0) ccw projected
  arc A278 (-67.174, -140.2423) -> (-67.698, -144.9723) centre (-37.3317, -145.9421) ccw projected
  arc A279 (-67.698, -144.9723) -> (-66.2715, -145.63) centre (0, 0) ccw projected
  arc A280 (-66.2715, -145.63) -> (-63.015, -142.1596) centre (-86.7302, -123.1691) ccw projected
  arc A281 (-63.015, -142.1596) -> (-61.6164, -142.7714) centre (0, 0) ccw projected
  arc A282 (-61.6164, -142.7714) -> (-61.9542, -147.5184) centre (-31.5733, -147.2952) ccw projected
  arc A283 (-61.9542, -147.5184) -> (-60.503, -148.1195) centre (0, 0) ccw projected
  arc A284 (-60.503, -148.1195) -> (-57.3853, -144.524) centre (-81.8277, -126.4791) ccw projected
  arc A285 (-57.3853, -144.524) -> (-55.9637, -145.0804) centre (0, 0) ccw projected
  arc A286 (-55.9637, -145.0804) -> (-56.1149, -149.837) centre (-25.7662, -148.4212) ccw projected
  arc A287 (-56.1149, -149.837) -> (-54.6412, -150.3806) centre (0, 0) ccw projected
  arc A288 (-54.6412, -150.3806) -> (-51.6671, -146.6655) centre (-76.7991, -129.5942) ccw projected
  arc A289 (-51.6671, -146.6655) -> (-50.2247, -147.1657) centre (0, 0) ccw projected
  arc A290 (-50.2247, -147.1657) -> (-50.1891, -151.9245) centre (-19.9193, -149.3183) ccw projected
  arc A291 (-50.1891, -151.9245) -> (-48.6952, -152.4099) centre (0, 0) ccw projected
  arc A292 (-48.6952, -152.4099) -> (-45.8692, -148.5809) centre (-71.6521, -132.5094) ccw projected
  arc A293 (-45.8692, -148.5809) -> (-44.4083, -149.024) centre (0, 0) ccw projected
  arc A294 (-44.4083, -149.024) -> (-44.1859, -153.7778) centre (-14.0418, -149.9853) ccw projected
  arc A295 (-44.1859, -153.7778) -> (-42.674, -154.2042) centre (0, 0) ccw projected
  arc A296 (-42.674, -154.2042) -> (-40.0005, -150.2671) centre (-66.3945, -135.2203) ccw projected
  arc A297 (-40.0005, -150.2671) -> (-38.5234, -150.6526) centre (0, 0) ccw projected
  arc A298 (-38.5234, -150.6526) -> (-38.1145, -155.394) centre (-8.1425, -150.4209) ccw projected
  arc A299 (-38.1145, -155.394) -> (-36.5871, -155.7607) centre (0, 0) ccw projected
  arc A300 (-36.5871, -155.7607) -> (-34.0702, -151.7217) centre (-61.0346, -137.7226) ccw projected
  arc A301 (-34.0702, -151.7217) -> (-32.5791, -152.0488) centre (0, 0) ccw projected
  arc A302 (-32.5791, -152.0488) -> (-31.9844, -156.7705) centre (-2.2308, -150.6246) ccw projected
  arc A303 (-31.9844, -156.7705) -> (-30.4438, -157.077) centre (0, 0) ccw projected
  arc A304 (-30.4438, -157.077) -> (-28.0874, -152.9423) centre (-55.5806, -140.0127) ccw projected
  arc A305 (-28.0874, -152.9423) -> (-26.5846, -153.2107) centre (0, 0) ccw projected
  arc A306 (-26.5846, -153.2107) -> (-25.8049, -157.9054) centre (3.6845, -150.5961) ccw projected
  arc A307 (-25.8049, -157.9054) -> (-24.2535, -158.1511) centre (0, 0) ccw projected
  arc A308 (-24.2535, -158.1511) -> (-22.0613, -153.9271) centre (-50.0409, -142.0868) ccw projected
  arc A309 (-22.0613, -153.9271) -> (-20.5491, -154.1363) centre (0, 0) ccw projected
  arc A310 (-20.5491, -154.1363) -> (-19.5857, -158.7967) centre (9.594, -150.3353) ccw projected
  arc A311 (-19.5857, -158.7967) -> (-18.0258, -158.9814) centre (0, 0) ccw projected
  arc A312 (-18.0258, -158.9814) -> (-16.0011, -154.6745) centre (-44.424, -143.9419) ccw projected
  arc A313 (-16.0011, -154.6745) -> (-14.4819, -154.8242) centre (0, 0) ccw projected
  arc A314 (-14.4819, -154.8242) -> (-13.3363, -159.4432) centre (15.4887, -149.8427) ccw projected
  arc A315 (-13.3363, -159.4432) -> (-11.7703, -159.5665) centre (0, 0) ccw projected
  arc A316 (-11.7703, -159.5665) -> (-9.9163, -155.1835) centre (-38.7386, -145.575) ccw projected
  arc A317 (-9.9163, -155.1835) -> (-8.3923, -155.2734) centre (0, 0) ccw projected
  arc A318 (-8.3923, -155.2734) -> (-7.0663, -159.8439) centre (21.3596, -149.1191) ccw projected
  arc A319 (-7.0663, -159.8439) -> (-5.4967, -159.9056) centre (0, 0) ccw projected
  arc A320 (-5.4967, -159.9056) -> (-3.8162, -155.4532) centre (-32.9935, -146.9836) ccw projected
  arc A321 (-3.8162, -155.4532) -> (-2.2898, -155.4831) centre (0, 0) ccw projected
  arc A322 (-2.2898, -155.4831) -> (-0.7854, -159.9981) centre (27.1975, -148.1656) ccw projected
  arc A323 (-0.7854, -159.9981) -> (0.7854, -159.9981) centre (0, 0) ccw projected
  arc A324 (0.7854, -159.9981) -> (2.2898, -155.4831) centre (-27.1975, -148.1656) ccw projected
  arc A325 (2.2898, -155.4831) -> (3.8162, -155.4532) centre (0, 0) ccw projected
  arc A326 (3.8162, -155.4532) -> (5.4967, -159.9056) centre (32.9935, -146.9836) ccw projected
  arc A327 (5.4967, -159.9056) -> (7.0663, -159.8439) centre (0, 0) ccw projected
  arc A328 (7.0663, -159.8439) -> (8.3923, -155.2734) centre (-21.3596, -149.1191) ccw projected
  arc A329 (8.3923, -155.2734) -> (9.9163, -155.1835) centre (0, 0) ccw projected
  arc A330 (9.9163, -155.1835) -> (11.7703, -159.5665) centre (38.7386, -145.575) ccw projected
  arc A331 (11.7703, -159.5665) -> (13.3363, -159.4432) centre (0, 0) ccw projected
  arc A332 (13.3363, -159.4432) -> (14.4819, -154.8242) centre (-15.4887, -149.8427) ccw projected
  arc A333 (14.4819, -154.8242) -> (16.0011, -154.6745) centre (0, 0) ccw projected
  arc A334 (16.0011, -154.6745) -> (18.0258, -158.9814) centre (44.424, -143.9419) ccw projected
  arc A335 (18.0258, -158.9814) -> (19.5857, -158.7967) centre (0, 0) ccw projected
  arc A336 (19.5857, -158.7967) -> (20.5491, -154.1363) centre (-9.594, -150.3353) ccw projected
  arc A337 (20.5491, -154.1363) -> (22.0613, -153.9271) centre (0, 0) ccw projected
  arc A338 (22.0613, -153.9271) -> (24.2535, -158.1511) centre (50.0409, -142.0868) ccw projected
  arc A339 (24.2535, -158.1511) -> (25.8049, -157.9054) centre (0, 0) ccw projected
  arc A340 (25.8049, -157.9054) -> (26.5846, -153.2107) centre (-3.6845, -150.5961) ccw projected
  arc A341 (26.5846, -153.2107) -> (28.0874, -152.9423) centre (0, 0) ccw projected
  arc A342 (28.0874, -152.9423) -> (30.4438, -157.077) centre (55.5806, -140.0127) ccw projected
  arc A343 (30.4438, -157.077) -> (31.9844, -156.7705) centre (0, 0) ccw projected
  arc A344 (31.9844, -156.7705) -> (32.5791, -152.0488) centre (2.2308, -150.6246) ccw projected
  arc A345 (32.5791, -152.0488) -> (34.0702, -151.7217) centre (0, 0) ccw projected
  arc A346 (34.0702, -151.7217) -> (36.5871, -155.7607) centre (61.0346, -137.7226) ccw projected
  arc A347 (36.5871, -155.7607) -> (38.1145, -155.394) centre (0, 0) ccw projected
  arc A348 (38.1145, -155.394) -> (38.5234, -150.6526) centre (8.1425, -150.4209) ccw projected
  arc A349 (38.5234, -150.6526) -> (40.0005, -150.2671) centre (0, 0) ccw projected
  arc A350 (40.0005, -150.2671) -> (42.674, -154.2042) centre (66.3945, -135.2203) ccw projected
  arc A351 (42.674, -154.2042) -> (44.1859, -153.7778) centre (0, 0) ccw projected
  arc A352 (44.1859, -153.7778) -> (44.4083, -149.024) centre (14.0418, -149.9853) ccw projected
  arc A353 (44.4083, -149.024) -> (45.8692, -148.5809) centre (0, 0) ccw projected
  arc A354 (45.8692, -148.5809) -> (48.6952, -152.4099) centre (71.6521, -132.5094) ccw projected
  arc A355 (48.6952, -152.4099) -> (50.1891, -151.9245) centre (0, 0) ccw projected
  arc A356 (50.1891, -151.9245) -> (50.2247, -147.1657) centre (19.9193, -149.3183) ccw projected
  arc A357 (50.2247, -147.1657) -> (51.6671, -146.6655) centre (0, 0) ccw projected
  arc A358 (51.6671, -146.6655) -> (54.6412, -150.3806) centre (76.7991, -129.5942) ccw projected
  arc A359 (54.6412, -150.3806) -> (56.1149, -149.837) centre (0, 0) ccw projected
  arc A360 (56.1149, -149.837) -> (55.9637, -145.0804) centre (25.7662, -148.4212) ccw projected
  arc A361 (55.9637, -145.0804) -> (57.3853, -144.524) centre (0, 0) ccw projected
  arc A362 (57.3853, -144.524) -> (60.503, -148.1195) centre (81.8277, -126.4791) ccw projected
  arc A363 (60.503, -148.1195) -> (61.9542, -147.5184) centre (0, 0) ccw projected
  arc A364 (61.9542, -147.5184) -> (61.6164, -142.7714) centre (31.5733, -147.2952) ccw projected
  arc A365 (61.6164, -142.7714) -> (63.015, -142.1596) centre (0, 0) ccw projected
  arc A366 (63.015, -142.1596) -> (66.2715, -145.63) centre (86.7302, -123.1691) ccw projected
  arc A367 (66.2715, -145.63) -> (67.698, -144.9723) centre (0, 0) ccw projected
  arc A368 (67.698, -144.9723) -> (67.174, -140.2423) centre (37.3317, -145.9421) ccw projected
  arc A369 (67.174, -140.2423) -> (68.5476, -139.5761) centre (0, 0) ccw projected
  arc A370 (68.5476, -139.5761) -> (71.9378, -142.9159) centre (91.4989, -119.6691) ccw projected
  arc A371 (71.9378, -142.9159) -> (73.3374, -142.2028) centre (0, 0) ccw projected
  arc A372 (73.3374, -142.2028) -> (72.6281, -137.4969) centre (43.0326, -144.3639) ccw projected
  arc A373 (72.6281, -137.4969) -> (73.9745, -136.7773) centre (0, 0) ccw projected
  arc A374 (73.9745, -136.7773) -> (77.4932, -139.9814) centre (96.1266, -115.9846) ccw projected
  arc A375 (77.4932, -139.9814) -> (78.8637, -139.2139) centre (0, 0) ccw projected
  arc A376 (78.8637, -139.2139) -> (77.9702, -134.5396) centre (48.6671, -142.5632) ccw projected
  arc A377 (77.9702, -134.5396) -> (79.2873, -133.7676) centre (0, 0) ccw projected
  arc A378 (79.2873, -133.7676) -> (82.9291, -136.8312) centre (100.606, -112.1213) ccw projected
  arc A379 (82.9291, -136.8312) -> (84.2684, -136.0104) centre (0, 0) ccw projected
  arc A380 (84.2684, -136.0104) -> (83.1921, -131.3747) centre (54.2266, -140.5426) ccw projected
  arc A381 (83.1921, -131.3747) -> (84.4779, -130.5517) centre (0, 0) ccw projected
  arc A382 (84.4779, -130.5517) -> (88.2371, -133.4699) centre (104.9303, -108.0851) ccw projected
  arc A383 (88.2371, -133.4699) -> (89.5432, -132.5972) centre (0, 0) ccw projected
  arc A384 (89.5432, -132.5972) -> (88.2857, -128.0073) centre (59.7025, -138.3053) ccw projected
  arc A385 (88.2857, -128.0073) -> (89.5382, -127.1344) centre (0, 0) ccw projected
  arc A386 (89.5382, -127.1344) -> (93.4091, -129.9028) centre (109.0928, -103.8822) ccw projected
  arc A387 (93.4091, -129.9028) -> (94.6799, -128.9795) centre (0, 0) ccw projected
  arc A388 (94.6799, -128.9795) -> (93.2432, -124.4426) centre (65.0863, -135.8548) ccw projected
  arc A389 (93.2432, -124.4426) -> (94.4604, -123.5212) centre (0, 0) ccw projected
  arc A390 (94.4604, -123.5212) -> (98.4371, -126.1354) centre (113.0871, -99.5191) ccw projected
  arc A391 (98.4371, -126.1354) -> (99.6706, -125.163) centre (0, 0) ccw projected
  arc A392 (99.6706, -125.163) -> (98.0569, -120.6859) centre (70.3698, -133.1948) ccw projected
  arc A393 (98.0569, -120.6859) -> (99.237, -119.7174) centre (0, 0) ccw projected
  arc A394 (99.237, -119.7174) -> (103.3132, -122.1736) centre (116.907, -95.0026) ccw projected
  arc A395 (103.3132, -122.1736) -> (104.5077, -121.1534) centre (0, 0) ccw projected
  arc A396 (104.5077, -121.1534) -> (102.7194, -116.7432) centre (75.5447, -130.3294) ccw projected
  arc A397 (102.7194, -116.7432) -> (103.8606, -115.7291) centre (0, 0) ccw projected
  arc A398 (103.8606, -115.7291) -> (108.0301, -118.0233) centre (120.5467, -90.3396) ccw projected
  arc A399 (108.0301, -118.0233) -> (109.1835, -116.9571) centre (0, 0) ccw projected
  arc A400 (109.1835, -116.9571) -> (107.2236, -112.6204) centre (80.6032, -127.263) ccw projected
  arc A401 (107.2236, -112.6204) -> (108.324, -111.5623) centre (0, 0) ccw projected
  arc A402 (108.324, -111.5623) -> (112.5804, -113.6911) centre (124.0004, -85.5374) ccw projected
  arc A403 (112.5804, -113.6911) -> (113.6911, -112.5804) centre (0, 0) ccw projected
  arc A404 (113.6911, -112.5804) -> (111.5623, -108.324) centre (85.5374, -124.0004) ccw projected
  arc A405 (111.5623, -108.324) -> (112.6204, -107.2236) centre (0, 0) ccw projected
  arc A406 (112.6204, -107.2236) -> (116.9571, -109.1835) centre (127.263, -80.6032) ccw projected
  arc A407 (116.9571, -109.1835) -> (118.0233, -108.0301) centre (0, 0) ccw projected
  arc A408 (118.0233, -108.0301) -> (115.7291, -103.8606) centre (90.3396, -120.5467) ccw projected
  arc A409 (115.7291, -103.8606) -> (116.7432, -102.7194) centre (0, 0) ccw projected
  arc A410 (116.7432, -102.7194) -> (121.1534, -104.5077) centre (130.3294, -75.5447) ccw projected
  arc A411 (121.1534, -104.5077) -> (122.1736, -103.3132) centre (0, 0) ccw projected
  arc A412 (122.1736, -103.3132) -> (119.7174, -99.237) centre (95.0026, -116.907) ccw projected
  arc A413 (119.7174, -99.237) -> (120.6859, -98.0569) centre (0, 0) ccw projected
  arc A414 (120.6859, -98.0569) -> (125.163, -99.6706) centre (133.1948, -70.3698) ccw projected
  arc A415 (125.163, -99.6706) -> (126.1354, -98.4371) centre (0, 0) ccw projected
  arc A416 (126.1354, -98.4371) -> (123.5212, -94.4604) centre (99.5191, -113.0871) ccw projected
  arc A417 (123.5212, -94.4604) -> (124.4426, -93.2432) centre (0, 0) ccw projected
  arc A418 (124.4426, -93.2432) -> (128.9795, -94.6799) centre (135.8548, -65.0863) ccw projected
  arc A419 (128.9795, -94.6799) -> (129.9028, -93.4091) centre (0, 0) ccw projected
  arc A420 (129.9028, -93.4091) -> (127.1344, -89.5382) centre (103.8822, -109.0928) ccw projected
  arc A421 (127.1344, -89.5382) -> (128.0073, -88.2857) centre (0, 0) ccw projected
  arc A422 (128.0073, -88.2857) -> (132.5972, -89.5432) centre (138.3053, -59.7025) ccw projected
  arc A423 (132.5972, -89.5432) -> (133.4699, -88.2371) centre (0, 0) ccw projected
  arc A424 (133.4699, -88.2371) -> (130.5517, -84.4779) centre (108.0851, -104.9303) ccw projected
  arc A425 (130.5517, -84.4779) -> (131.3747, -83.1921) centre (0, 0) ccw projected
  arc A426 (131.3747, -83.1921) -> (136.0104, -84.2684) centre (140.5426, -54.2266) ccw projected
  arc A427 (136.0104, -84.2684) -> (136.8312, -82.9291) centre (0, 0) ccw projected
  arc A428 (136.8312, -82.9291) -> (133.7676, -79.2873) centre (112.1213, -100.606) ccw projected
  arc A429 (133.7676, -79.2873) -> (134.5396, -77.9702) centre (0, 0) ccw projected
  arc A430 (134.5396, -77.9702) -> (139.2139, -78.8637) centre (142.5632, -48.6671) ccw projected
  arc A431 (139.2139, -78.8637) -> (139.9814, -77.4932) centre (0, 0) ccw projected
  arc A432 (139.9814, -77.4932) -> (136.7773, -73.9745) centre (115.9846, -96.1266) ccw projected
  arc A433 (136.7773, -73.9745) -> (137.4969, -72.6281) centre (0, 0) ccw projected
  arc A434 (137.4969, -72.6281) -> (142.2028, -73.3374) centre (144.3639, -43.0326) ccw projected
  arc A435 (142.2028, -73.3374) -> (142.9159, -71.9378) centre (0, 0) ccw projected
  arc A436 (142.9159, -71.9378) -> (139.5761, -68.5476) centre (119.6691, -91.4989) ccw projected
  arc A437 (139.5761, -68.5476) -> (140.2423, -67.174) centre (0, 0) ccw projected
  arc A438 (140.2423, -67.174) -> (144.9723, -67.698) centre (145.9421, -37.3317) ccw projected
  arc A439 (144.9723, -67.698) -> (145.63, -66.2715) centre (0, 0) ccw projected
  arc A440 (145.63, -66.2715) -> (142.1596, -63.015) centre (123.1691, -86.7302) ccw projected
  arc A441 (142.1596, -63.015) -> (142.7714, -61.6164) centre (0, 0) ccw projected
  arc A442 (142.7714, -61.6164) -> (147.5184, -61.9542) centre (147.2952, -31.5733) ccw projected
  arc A443 (147.5184, -61.9542) -> (148.1195, -60.503) centre (0, 0) ccw projected
  arc A444 (148.1195, -60.503) -> (144.524, -57.3853) centre (126.4791, -81.8277) ccw projected
  arc A445 (144.524, -57.3853) -> (145.0804, -55.9637) centre (0, 0) ccw projected
  arc A446 (145.0804, -55.9637) -> (149.837, -56.1149) centre (148.4212, -25.7662) ccw projected
  arc A447 (149.837, -56.1149) -> (150.3806, -54.6412) centre (0, 0) ccw projected
  arc A448 (150.3806, -54.6412) -> (146.6655, -51.6671) centre (129.5942, -76.7991) ccw projected
  arc A449 (146.6655, -51.6671) -> (147.1657, -50.2247) centre (0, 0) ccw projected
  arc A450 (147.1657, -50.2247) -> (151.9245, -50.1891) centre (149.3183, -19.9193) ccw projected
  arc A451 (151.9245, -50.1891) -> (152.4099, -48.6952) centre (0, 0) ccw projected
  arc A452 (152.4099, -48.6952) -> (148.5809, -45.8692) centre (132.5094, -71.6521) ccw projected
  arc A453 (148.5809, -45.8692) -> (149.024, -44.4083) centre (0, 0) ccw projected
  arc A454 (149.024, -44.4083) -> (153.7778, -44.1859) centre (149.9853, -14.0418) ccw projected